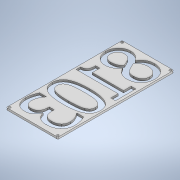
# Autodesk Inventor part: number_plate
Saved by Autodesk Inventor 2022 (Build 260153000, 153)
## iProperties
Created: 2021-07-20
Part Number: number_plate
Material: Generic
Document SubType Name: Modeling
Designer: gfellows
Density: 1 g/cm^3
Appearance: Default
Author: gfellows
Autodesk Inventor part; units mm, degrees
ref_plane "YZ Plane" through (0, 0, 0) normal (1, 0, 0) x (0, 1, 0)
ref_plane "XZ Plane" through (0, 0, 0) normal (0, 1, 0) x (-1, 0, 0)
ref_plane "XY Plane" through (0, 0, 0) normal (0, 0, 1) x (1, 0, 0)
sketch "Sketch1" plane through (0, 0, 0) normal (0, 1, 0) x (-1, 0, 0)
  line L0 (0, 0) -> (81.5, 0)
  line L1 (81.5, 0) -> (81.5, -183.1)
  line L2 (81.5, -183.1) -> (0, -183.1)
  line L3 (0, -183.1) -> (0, 0)
  line L4 (0, 0) -> (81.5, -183.1) construction
  line L5 (78.85, -2.65) -> (2.65, -2.65) construction
  line L6 (2.65, -2.65) -> (2.65, -180.45) construction
  line L7 (2.65, -180.45) -> (78.85, -180.45) construction
  line L8 (78.85, -180.45) -> (78.85, -2.65) construction
  line L9 (78.85, -2.65) -> (2.65, -180.45) construction
  line L10 (2.65, -2.65) -> (78.85, -180.45) construction
  circle A0 centre (78.85, -2.65) radius 1.65
  circle A1 centre (78.85, -180.45) radius 1.65
  circle A2 centre (2.65, -180.45) radius 1.65
  circle A3 centre (2.65, -2.65) radius 1.65
  point P0 (40.75, -91.55)
  dimension "d0" = 81.5
  dimension "d1" = 183.1
  dimension "d2" = 76.2
  dimension "d3" = 177.8
  dimension "d4" = 3.3
  dimension "d5" = 3.3
  dimension "d6" = 3.3
  dimension "d7" = 3.3
  constraints: 22 end point, 4 centre point, 4 coincident, 4 parallel, 3 midpoint, 2 horizontal, 2 perpendicular
  measures "d0" distance of L1.end L2.end
  measures "d1" distance of L2.end L0.start
  measures "d2" distance of L7.end L6.end
  measures "d3" distance of L6.end L5.end
  measures "d4" diameter of A0
  measures "d5" diameter of A1
  measures "d6" diameter of A2
  measures "d7" diameter of A3
extrude "Extrusion1" add sketch "Sketch1" along normal blind 3.175
fillet "Fillet1" radius 1.5 4 edges at (0, 1.5875, 0) (0, 1.5875, -183.1) (-81.5, 1.5875, -183.1) (-81.5, 1.5875, 0)
sketch "Sketch3" plane through (0, 0, 0) normal (0, -1, 0) x (1, 0, 0)
  arc A0 (-80, 0) -> (-81.5, -1.5) centre (-80, -1.5) ccw projected
  line L0 (-81.5, -181.6) -> (-81.5, -1.5) projected
  arc A1 (-81.5, -181.6) -> (-80, -183.1) centre (-80, -181.6) ccw projected
  line L1 (-1.5, -183.1) -> (-80, -183.1) projected
  arc A2 (-1.5, -183.1) -> (0, -181.6) centre (-1.5, -181.6) ccw projected
  line L2 (0, -1.5) -> (0, -181.6) projected
  arc A3 (0, -1.5) -> (-1.5, 0) centre (-1.5, -1.5) ccw projected
  line L3 (-80, 0) -> (-1.5, 0) projected
  circle A4 centre (-2.65, -2.65) radius 1.65 projected
  circle A5 centre (-2.65, -180.45) radius 1.65 projected
  circle A6 centre (-78.85, -180.45) radius 1.65 projected
  circle A7 centre (-78.85, -2.65) radius 1.65 projected
  circle A8 centre (-2.65, -180.45) radius 1.65 construction
  line L4 (-4.3, -180.45) -> (-4.3, -2.65) construction
  spline S0 degree 2 poles (-2.6286, -155.5584) (-2.6286, -160.5129) (-5.9117, -168.631) (-8.956, -171.4962) knots 0 0 0 1 2 2 2
  spline S1 degree 2 poles (-8.956, -171.4962) (-11.9406, -174.3017) (-20.0587, -177.1669) (-24.655, -177.1669) knots 0 0 0 1 2 2 2
  spline S2 degree 2 poles (-24.655, -177.1669) (-30.6242, -177.1669) (-40.6525, -171.4365) (-43.6371, -165.9448) knots 0 0 0 1 2 2 2
  line L5 (-43.6371, -165.9448) -> (-43.9355, -165.9448)
  spline S3 degree 2 poles (-43.9355, -165.9448) (-47.0992, -170.8396) (-54.6204, -175.5553) (-60.2315, -175.5553) knots 0 0 0 1 2 2 2
  spline S4 degree 2 poles (-60.2315, -175.5553) (-68.5287, -175.5553) (-79.6314, -164.2735) (-79.6314, -155.6181) knots 0 0 0 1 2 2 2
  spline S5 degree 2 poles (-79.6314, -155.6181) (-79.6314, -146.5449) (-69.1256, -135.681) (-60.8881, -135.681) knots 0 0 0 1 2 2 2
  spline S6 degree 2 poles (-60.8881, -135.681) (-55.9336, -135.681) (-46.2635, -140.8742) (-43.5177, -145.7689) knots 0 0 0 1 2 2 2
  line L6 (-43.5177, -145.7689) -> (-43.2192, -145.7689)
  spline S7 degree 2 poles (-43.2192, -145.7689) (-40.2346, -139.9788) (-31.639, -134.0096) (-24.8341, -134.0096) knots 0 0 0 1 2 2 2
  spline S8 degree 2 poles (-24.8341, -134.0096) (-15.4027, -134.0096) (-2.6286, -146.3061) (-2.6286, -155.5584) knots 0 0 0 1 2 2 2
  spline S9 degree 2 poles (-23.879, -143.1425) (-28.4156, -143.1425) (-33.7879, -146.3658) (-36.5337, -150.9024) knots 0 0 0 1 2 2 2
  spline S10 degree 2 poles (-36.5337, -150.9024) (-37.4888, -152.4544) (-39.6974, -157.4686) (-41.13, -160.6322) knots 0 0 0 1 2 2 2
  spline S11 degree 2 poles (-41.13, -160.6322) (-38.4439, -164.2735) (-30.4451, -168.2131) (-25.3713, -168.2131) knots 0 0 0 1 2 2 2
  spline S12 degree 2 poles (-25.3713, -168.2131) (-18.6858, -168.2131) (-9.9707, -160.9904) (-9.9707, -155.4987) knots 0 0 0 1 2 2 2
  spline S13 degree 2 poles (-9.9707, -155.4987) (-9.9707, -149.8877) (-17.4323, -143.1425) (-23.879, -143.1425) knots 0 0 0 1 2 2 2
  spline S14 degree 2 poles (-60.7687, -144.396) (-65.7231, -144.396) (-72.3489, -150.3652) (-72.3489, -155.6181) knots 0 0 0 1 2 2 2
  spline S15 degree 2 poles (-72.3489, -155.6181) (-72.3489, -160.5129) (-66.4394, -166.6611) (-61.3656, -166.6611) knots 0 0 0 1 2 2 2
  spline S16 degree 2 poles (-61.3656, -166.6611) (-57.7244, -166.6611) (-52.6506, -163.4975) (-50.621, -160.3338) knots 0 0 0 1 2 2 2
  spline S17 degree 2 poles (-50.621, -160.3338) (-49.7853, -158.9609) (-46.8604, -153.2901) (-46.0247, -151.0218) knots 0 0 0 1 2 2 2
  spline S18 degree 2 poles (-46.0247, -151.0218) (-49.3078, -147.1418) (-56.2918, -144.396) (-60.7687, -144.396) knots 0 0 0 1 2 2 2
  line L7 (-4.3, -95.3765) -> (-4.3, -127.6699)
  line L8 (-4.3, -127.6699) -> (-11.8212, -127.6699)
  line L9 (-11.8212, -127.6699) -> (-11.8212, -115.6718)
  line L10 (-11.8212, -115.6718) -> (-61.1865, -115.6718)
  line L11 (-61.1865, -115.6718) -> (-61.1865, -127.6699)
  line L12 (-61.1865, -127.6699) -> (-67.9317, -127.6699)
  spline S19 degree 2 poles (-67.9317, -127.6699) (-67.9317, -120.865) (-72.2296, -114.4182) (-78.1988, -114.0004) knots 0 0 0 1 2 2 2
  line L13 (-78.1988, -114.0004) -> (-78.1988, -107.1358)
  line L14 (-78.1988, -107.1358) -> (-11.8212, -107.1358)
  line L15 (-11.8212, -107.1358) -> (-11.8212, -95.3765)
  line L16 (-11.8212, -95.3765) -> (-4.3, -95.3765)
  spline S20 degree 2 poles (-41.13, -49.0431) (-21.3122, -49.0431) (-2.748, -59.4295) (-2.748, -70.1741) knots 0 0 0 1 2 2 2
  spline S21 degree 2 poles (-2.748, -70.1741) (-2.748, -81.1574) (-21.6704, -91.3648) (-41.0703, -91.3648) knots 0 0 0 1 2 2 2
  spline S22 degree 2 poles (-41.0703, -91.3648) (-61.0075, -91.3648) (-79.4523, -80.9783) (-79.4523, -70.1741) knots 0 0 0 1 2 2 2
  spline S23 degree 2 poles (-79.4523, -70.1741) (-79.4523, -59.2504) (-60.3508, -49.0431) (-41.13, -49.0431) knots 0 0 0 1 2 2 2
  spline S24 degree 2 poles (-18.6858, -60.3846) (-22.327, -59.131) (-33.5491, -58.0566) (-41.13, -58.0566) knots 0 0 0 1 2 2 2
  spline S25 degree 2 poles (-41.13, -58.0566) (-48.7109, -58.0566) (-59.8733, -59.131) (-63.6339, -60.4443) knots 0 0 0 1 2 2 2
  spline S26 degree 2 poles (-63.6339, -60.4443) (-67.3945, -61.8172) (-71.2745, -66.4732) (-71.2745, -70.1741) knots 0 0 0 1 2 2 2
  spline S27 degree 2 poles (-71.2745, -70.1741) (-71.2745, -73.875) (-67.3945, -78.6503) (-63.5145, -80.0233) knots 0 0 0 1 2 2 2
  spline S28 degree 2 poles (-63.5145, -80.0233) (-59.7539, -81.3962) (-48.293, -82.3512) (-41.0703, -82.3512) knots 0 0 0 1 2 2 2
  spline S29 degree 2 poles (-41.0703, -82.3512) (-33.3103, -82.3512) (-22.9239, -81.5156) (-18.8649, -80.083) knots 0 0 0 1 2 2 2
  spline S30 degree 2 poles (-18.8649, -80.083) (-15.0446, -78.7697) (-10.9258, -74.0541) (-10.9258, -70.1741) knots 0 0 0 1 2 2 2
  spline S31 degree 2 poles (-10.9258, -70.1741) (-10.9258, -66.5329) (-14.8058, -61.7575) (-18.6858, -60.3846) knots 0 0 0 1 2 2 2
  spline S32 degree 2 poles (-70.976, -29.6905) (-70.976, -32.0782) (-69.6628, -36.8536) (-68.648, -39.1815) knots 0 0 0 1 2 2 2
  spline S33 degree 2 poles (-68.648, -39.1815) (-67.6333, -41.3305) (-65.4844, -44.4344) (-64.5293, -45.688) knots 0 0 0 1 2 2 2
  line L17 (-64.5293, -45.688) -> (-64.5293, -46.2252)
  line L18 (-64.5293, -46.2252) -> (-74.9754, -46.2252)
  spline S34 degree 2 poles (-74.9754, -46.2252) (-76.7065, -43.36) (-79.512, -33.4511) (-79.512, -28.9742) knots 0 0 0 1 2 2 2
  spline S35 degree 2 poles (-79.512, -28.9742) (-79.512, -24.4973) (-77.4825, -17.7521) (-75.3336, -15.0659) knots 0 0 0 1 2 2 2
  spline S36 degree 2 poles (-75.3336, -15.0659) (-73.0056, -12.141) (-66.2604, -9.1564) (-61.7238, -9.1564) knots 0 0 0 1 2 2 2
  spline S37 degree 2 poles (-61.7238, -9.1564) (-55.6352, -9.1564) (-46.4426, -16.3195) (-45.2488, -21.3336) knots 0 0 0 1 2 2 2
  line L19 (-45.2488, -21.3336) -> (-44.5324, -21.3336)
  spline S38 degree 2 poles (-44.5324, -21.3336) (-44.0549, -19.2444) (-41.906, -14.5287) (-39.7571, -12.4395) knots 0 0 0 1 2 2 2
  spline S39 degree 2 poles (-39.7571, -12.4395) (-37.6679, -10.41) (-30.9824, -7.8432) (-26.1473, -7.8432) knots 0 0 0 1 2 2 2
  spline S40 degree 2 poles (-26.1473, -7.8432) (-21.1929, -7.8432) (-12.7763, -10.8875) (-9.5529, -13.693) knots 0 0 0 1 2 2 2
  spline S41 degree 2 poles (-9.5529, -13.693) (-6.2101, -16.6179) (-2.748, -24.7958) (-2.748, -29.989) knots 0 0 0 1 2 2 2
  spline S42 degree 2 poles (-2.748, -29.989) (-2.748, -34.9434) (-5.4341, -44.7329) (-7.2846, -48.0757) knots 0 0 0 1 2 2 2
  line L20 (-7.2846, -48.0757) -> (-17.7307, -48.0757)
  line L21 (-17.7307, -48.0757) -> (-17.7307, -47.4787)
  spline S43 degree 2 poles (-17.7307, -47.4787) (-15.4624, -44.6732) (-11.284, -35.2419) (-11.284, -30.5262) knots 0 0 0 1 2 2 2
  spline S44 degree 2 poles (-11.284, -30.5262) (-11.284, -27.7804) (-13.1941, -22.3484) (-15.4027, -20.4979) knots 0 0 0 1 2 2 2
  spline S45 degree 2 poles (-15.4027, -20.4979) (-17.6113, -18.7072) (-22.8642, -16.8567) (-26.8636, -16.8567) knots 0 0 0 1 2 2 2
  spline S46 degree 2 poles (-26.8636, -16.8567) (-30.863, -16.8567) (-36.0562, -18.9459) (-37.5485, -20.7964) knots 0 0 0 1 2 2 2
  spline S47 degree 2 poles (-37.5485, -20.7964) (-39.0408, -22.7065) (-40.1749, -27.8401) (-40.1749, -30.8247) knots 0 0 0 1 2 2 2
  line L22 (-40.1749, -30.8247) -> (-40.1749, -34.5853)
  line L23 (-40.1749, -34.5853) -> (-48.3527, -34.5853)
  line L24 (-48.3527, -34.5853) -> (-48.3527, -31.6603)
  spline S48 degree 2 poles (-48.3527, -31.6603) (-48.3527, -25.6911) (-54.6801, -18.1699) (-60.709, -18.1699) knots 0 0 0 1 2 2 2
  spline S49 degree 2 poles (-60.709, -18.1699) (-63.5145, -18.1699) (-67.5139, -20.1398) (-68.7077, -21.6321) knots 0 0 0 1 2 2 2
  spline S50 degree 2 poles (-68.7077, -21.6321) (-69.9613, -23.3035) (-70.976, -27.3625) (-70.976, -29.6905) knots 0 0 0 1 2 2 2
  point P0 (0, 0)
  constraints: 3 vertical, 2 end point, 2 horizontal alignment, 2 other
extrude "Extrusion2" cut sketch "Sketch3" against normal through all contours S0 S1 S2 L5 S3 S4 S5 S6 L6 S7 S8 | L7 L8 L9 L10 L11 L12 S19 L13 L14 L15 L16 | S20 S21 S22 S23 | S32 S33 L17 L18 S34 S35 S36 S37 L19 S38 S39 S40 S41 S42 L20 L21 S43 S44 S45 S46 S47 L22 L23 L24 S48 S49 S50
body "Solid1"
